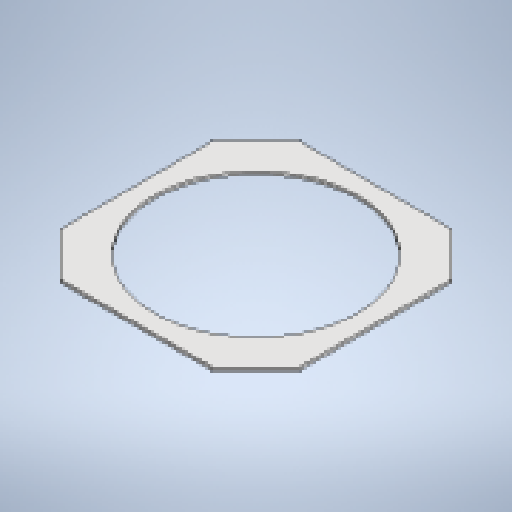
# Autodesk Inventor part: ANP 1453 BOTTOM DS reduce flange
Saved by Autodesk Inventor 2025 (Build 290162010, 162A)
## iProperties
Created: 2024-12-09
Part Number: ANP 1453 BOTTOM DS reduce flange
Material: Stainless Steel
Document SubType Name: Sheet Metal
Designer: user
Mass: 3269.02 g
Surface Area: 1007.63 cm^2
Volume: 408.627 cm^3
Density: 8 g/cm^3
Flat Pattern Width: 23.4853 cm
Flat Pattern Length: 23.4853 cm
Flat Pattern Area: 551.558 cm^2
Sheet Metal Rule: AISI304 3mm Die 32
Sheet Metal Width: 234,853 mm
Sheet Metal Length: 234,853 mm
Sheet Metal Area: 55155,844 mm^2
Appearance: Default
Wall_1_width: 150,000 mm
Wall_2_width: 60,000 mm
Author: user
Autodesk Inventor part; units mm, degrees
ref_plane "YZ Plane" through (0, 0, 0) normal (1, 0, 0) x (0, 1, 0)
ref_plane "XZ Plane" through (0, 0, 0) normal (0, 1, 0) x (-1, 0, 0)
ref_plane "XY Plane" through (0, 0, 0) normal (0, 0, 1) x (1, 0, 0)
sketch "Sketch1" plane through (0, 0, 0) normal (0, 0, 1) x (1, 0, 0)
  circle A0 centre (0, 0) radius 100
  line L0 (-117.4264, -75) -> (-117.4264, 75)
  line L1 (-117.4264, 75) -> (-75, 117.4264)
  line L2 (-75, 117.4264) -> (75, 117.4264)
  line L3 (75, 117.4264) -> (117.4264, 75)
  line L4 (117.4264, 75) -> (117.4264, -75)
  line L5 (117.4264, -75) -> (75, -117.4264)
  line L6 (75, -117.4264) -> (-75, -117.4264)
  line L7 (-75, -117.4264) -> (-117.4264, -75)
  point P0 (-117.4264, 0)
  point P1 (117.4264, 0)
  point P2 (0, 117.4264)
  point P3 (0, -117.4264)
  dimension "d22" = 200
  dimension "d33" = 150
  dimension "d35" = 60
  measures "d22" diameter of A0
  measures "d33" distance of L5.end L6.end
  measures "d35" distance of L6.end L0.start
extrude "Plate1" add sketch "Sketch1" along normal blind 3
equation "\"d33\" = Wall_1_width"
equation "\"d35\" = Wall_2_width"
equation "\"d2\" = Thickness"
equation "\"BendReliefWidth\" = Thickness"
equation "\"BendReliefDepth\" = 0.5 * Thickness"
equation "\"CornerReliefSize\" = 4 * Thickness"
equation "\"MinimumRemnant\" = 2 * Thickness"
equation "\"TransitionRadius\" = BendRadius"
equation "\"JacobiRadiusSize\" = BendRadius"
equation "\"GapSize\" = Thickness"
equation "\"Wall_1_width\" = 150"
equation "\"Wall_2_width\" = 60"
equation "\"Thickness\" = 3"
equation "\"BendRadius\" = 5"
body "Solid1"
